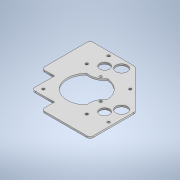
# Autodesk Inventor part: TopPlate2
Saved by Autodesk Inventor 2020 (Build 240168000, 168)
## iProperties
Created: 2019-05-28
Part Number: TopPlate2
Material: Generic
Document SubType Name: Modeling
Designer: Connor
Density: 1 g/cm^3
Appearance: Default
Author: Connor
Autodesk Inventor part; units mm, degrees
ref_plane "YZ Plane" through (0, 0, 0) normal (1, 0, 0) x (0, 1, 0)
ref_plane "XZ Plane" through (0, 0, 0) normal (0, 1, 0) x (-1, 0, 0)
ref_plane "XY Plane" through (0, 0, 0) normal (0, 0, 1) x (1, 0, 0)
sketch "Sketch1" plane through (0, 0, 0) normal (0, 1, 0) x (-1, 0, 0)
  line L0 (0, 0) -> (-165.1, 0)
  line L1 (-165.1, 0) -> (-165.1, -165.1)
  line L2 (-165.1, -165.1) -> (0, -165.1)
  line L3 (0, -165.1) -> (0, 0)
  circle A0 centre (-79.375, -79.375) radius 38.1
  line L4 (-25.4, -165.1) -> (-25.4, 0) construction
  line L5 (0, -25.4) -> (-165.1, -25.4) construction
  line L6 (0, 0) -> (-165.1, -165.1) construction
  circle A1 centre (-79.375, -79.375) radius 53.975 construction
  dimension "d0" = 76.2
  dimension "d3" = 25.4
  dimension "d4" = 25.4
  dimension "d5" = 107.95
  dimension "d25" = 165.1
  constraints: 14 end point, 7 point on line, 4 perpendicular, 2 centre point, 2 parallel, 1 coincident, 1 horizontal, 1 tangent
  measures "d0" diameter of A0
  measures "d3" distance between parallel lines of L0 L5
  measures "d4" distance between parallel lines of L3 L4
  measures "d5" diameter of A1
  measures "d25" distance between parallel lines of L0 L2
extrude "Extrusion1" add sketch "Sketch1" along normal blind 3.175
sketch "Sketch2" plane through (0, 3.175, 0) normal (0, 1, 0) x (1, 0, 0)
  circle A0 centre (79.375, 79.375) radius 38.1 construction
  circle A1 centre (79.375, 79.375) radius 60.325 construction
  line L0 (0, 165.1) -> (0, 0) construction
  arc A2 (184.15, 82.55) -> (82.55, 184.15) centre (82.55, 82.55) ccw construction
  line L1 (36.7188, 36.7188) -> (122.0312, 36.7188) construction
  line L2 (122.0312, 36.7188) -> (122.0312, 122.0312) construction
  line L3 (122.0312, 122.0312) -> (36.7188, 122.0312) construction
  line L4 (36.7188, 122.0312) -> (36.7188, 36.7188) construction
  dimension "d9" = 120.65
  constraints: 8 end point, 4 point on circle, 2 parallel, 2 perpendicular, 1 centre point, 1 coincident, 1 horizontal
  measures "d9" diameter of A1
hole "Hole1" at (36.7188, 3.175, -36.7188) at (122.0312, 3.175, -122.0312) at (122.0312, 3.175, -36.7188) at (36.7188, 3.175, -122.0312) direction (0, -1, 0) diameter 4.9784 end through all
sketch "Sketch3" plane through (0, 3.175, 0) normal (0, 1, 0) x (1, 0, 0)
  circle A0 centre (79.375, 79.375) radius 38.1 construction
  circle A1 centre (79.375, 79.375) radius 53.975 construction
  circle A2 centre (58.1423, 135.6764) radius 9.525
  line L0 (0, 0) -> (79.375, 79.375) construction
  circle A3 centre (135.6764, 58.1423) radius 9.525
  circle A4 centre (122.0312, 122.0312) radius 2.4892 construction
  circle A5 centre (58.1423, 135.6764) radius 24.13 construction
  line L1 (79.375, 79.375) -> (78.4947, 148.6394) construction
  circle A6 centre (78.4947, 148.6394) radius 11.1125
  circle A7 centre (148.6394, 78.4947) radius 11.1125
  circle A8 centre (58.1423, 135.6764) radius 25.4 construction
  circle A9 centre (122.0312, 122.0312) radius 4.7625 construction
  circle A10 centre (58.1423, 135.6764) radius 29.9974 construction
  circle A11 centre (36.7188, 122.0312) radius 2.4892 projected
  circle A12 centre (44.4971, 157.1) radius 2.4892
  circle A13 centre (122.0312, 36.7188) radius 2.4892
  circle A14 centre (157.1, 44.4971) radius 2.4892
  circle A15 centre (71.7875, 114.2529) radius 2.4892
  circle A16 centre (114.2529, 71.7875) radius 2.4892
  circle A17 centre (79.375, 79.375) radius 38.1 projected
  arc A18 (52.3602, 106.2416) -> (81.9214, 117.3898) centre (58.1423, 135.6764) ccw
  arc A19 (117.3898, 81.9214) -> (106.2416, 52.3602) centre (135.6764, 58.1423) ccw
  circle A20 centre (36.7188, 122.0312) radius 2.4892 projected
  line L2 (36.7188, 122.0312) -> (78.4947, 148.6394) construction
  point P0 (117.3898, 81.9214)
  point P1 (106.2416, 52.3602)
  dimension "d33" = 48.26
  dimension "d17" = 107.95
  dimension "d19" = 19.05
  dimension "d34" = 69.27
  dimension "d35" = 22.225
  dimension "d37" = 50.8
  dimension "d38" = 59.9948
  dimension "d39" = 9.525
  dimension "d52" = 4.9784
  dimension "d53" = 90
  dimension "d56" = 90
  constraints: 15 centre point, 11 point on circle, 8 symmetric about line, 7 coincident, 6 end point, 1 equal radius, 1 point on line, 9 other
  measures "d17" diameter of A1
  measures "d19" diameter of A2
  measures "d34" distance of L0.end L1.end
  measures "d35" diameter of A6
  measures "d37" diameter of A8
  measures "d38" diameter of A10
  measures "d39" diameter of A9
  measures "d52" diameter of A12
extrude "Extrusion5" cut sketch "Sketch3" against normal through all contours A2 | A3 | A6 | A7 | A12 | A14 | A15 A17 | A17 A15 | A17 A16 | A16 A17
extrude "Extrusion6" add sketch "Sketch3" against normal up to surface (3.175 mm away) contours A15 A17 A18 | A17 A16 A19
sketch "Sketch5" plane through (0, 3.175, 0) normal (0, 1, 0) x (1, 0, 0)
  line L0 (0, 165.1) -> (0, 0) projected
  line L1 (0, 0) -> (25.4, 0)
  line L2 (25.4, 0) -> (25.4, 69.85)
  line L3 (25.4, 69.85) -> (0, 69.85)
  line L4 (0, 69.85) -> (0, 0)
  line L5 (25.4, 0) -> (69.85, 0)
  line L6 (69.85, 0) -> (69.85, 25.4)
  line L7 (69.85, 25.4) -> (25.4, 25.4)
  line L8 (25.4, 25.4) -> (25.4, 0)
  dimension "d63" = 25.4
  dimension "d64" = 69.85
  dimension "d65" = 44.45
  dimension "d66" = 25.4
  constraints: 16 end point, 4 parallel, 2 horizontal, 2 perpendicular
  measures "d63" distance of L3.end L2.end
  measures "d64" distance of L2.end L1.end
  measures "d65" distance of L7.end L6.end
  measures "d66" distance of L6.end L5.end
extrude "Extrusion7" cut sketch "Sketch5" against normal up to surface (3.175 mm away)
chamfer "Chamfer3" distance 76.2 angle 45 1 edges at (165.1, 1.5875, -165.1)
fillet "Fillet6" radius 6.35 7 edges at (165.1, 1.5875, 0) (165.1, 1.5875, -88.9) (88.9, 1.5875, -165.1) (0, 1.5875, -165.1) (25.4, 1.5875, -25.4) (0, 1.5875, -69.85) (69.85, 1.5875, 0)
body "Solid1"
